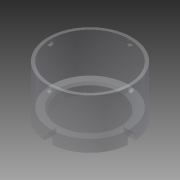
# Autodesk Inventor part: 13_1087_029
Saved by Autodesk Inventor 2014 (Build 180170000, 170)
## iProperties
Created: 2013-09-17
Part Number: 13_1087_029
Material: Allgemein
Document SubType Name: Modeling
Designer: vogel
Density: 1 g/cm^3
Appearance: Klar - hell
Author: vogel
Autodesk Inventor part; units mm, degrees
ref_plane "YZ Plane" through (0, 0, 0) normal (1, 0, 0) x (0, 1, 0)
ref_plane "XY Plane" through (0, 0, 0) normal (0, 0, 1) x (1, 0, 0)
sketch "Skizze1" plane through (0, 0, 0) normal (0, 0, 1) x (1, 0, 0)
  line L0 (-29.4, 0) -> (29.4, 0) projected
  line L1 (0, -29.4) -> (0, 29.4) projected
  circle A0 centre (0, 0) radius 21
  dimension "d0" = 42
  constraints: 1 centre point, 1 coincident
  measures "d0" diameter of A0
extrude "Extrusion1" add sketch "Skizze1" along normal blind 25
sketch "Skizze2" plane through (0, 0, 25) normal (0, 0, 1) x (1, 0, 0)
  circle A0 centre (0, 0) radius 21 projected
  circle A1 centre (0, 0) radius 19.5
  dimension "d3" = 39
  constraints: 1 centre point, 1 coincident
  measures "d3" diameter of A1
extrude "Extrusion2" cut sketch "Skizze2" against normal blind 20 contours A1
sketch "Skizze3" plane through (0, 0, 0) normal (0, 0, -1) x (-1, 0, 0)
  circle A0 centre (0, 0) radius 21 projected
  circle A1 centre (0, 0) radius 15
  dimension "d6" = 30
  constraints: 1 centre point, 1 coincident
  measures "d6" diameter of A1
extrude "Extrusion3" cut sketch "Skizze3" against normal through all contours A1
ref_plane "Arbeitsebene1" through (0, 21, 0) normal (0, 1, 0) x (-1, 0, 0)
sketch "Skizze5" plane through (0, 21, 0) normal (0, 1, 0) x (-1, 0, 0)
  line L0 (0, -5) -> (0, 30) projected
  line L1 (29.4, 0) -> (-29.4, 0) projected
  line L2 (21, 25) -> (-21, 25) projected
  point P0 (0, 0)
  point P1 (0, 23)
  dimension "d13" = 2
  constraints: 1 point on line
  measures "d13" distance from line of point (0, 23) L2
hole "Bohrung1" at (0, 21, 23) direction (0, -1, 0) diameter 2.4 end through all
pattern_circular "Runde Anordnung1" count 4 over 360 about axis through (0, 0, 0) along (0, 0, 1) of "Bohrung1"
chamfer "Fase1" distance 1 angle 45 1 edges at (15, 0, 5)
sketch "Skizze6" plane through (0, 21, 0) normal (0, 1, 0) x (-1, 0, 0)
  line L0 (29.4, 0) -> (-29.4, 0) projected
  line L1 (0, -5) -> (0, 30) projected
  line L2 (-2, 0) -> (2, 0)
  line L3 (2, 0) -> (2, 2)
  line L4 (0, 4) -> (0, 4)
  line L5 (-2, 2) -> (-2, 0)
  arc A0 (2, 2) -> (0, 4) centre (0, 2) ccw
  arc A1 (0, 4) -> (-2, 2) centre (0, 2) ccw
  point P0 (0, 0)
  dimension "d27" = 4
  dimension "d28" = 4
  dimension "d29" = 2
  constraints: 8 end point, 4 point on circle, 4 tangent, 2 centre point, 2 parallel, 1 concentric, 1 horizontal, 1 perpendicular, 1 point on line, 1 other
  measures "d27" distance between parallel lines of L0 L4
  measures "d28" distance between parallel lines of L3 L5
  measures "d29" radius of A0
extrude "Extrusion6" cut sketch "Skizze6" against normal through all
pattern_circular "Runde Anordnung2" count 4 over 360 about axis through (0, 0, 0) along (0, 0, 1) of "Extrusion6"
